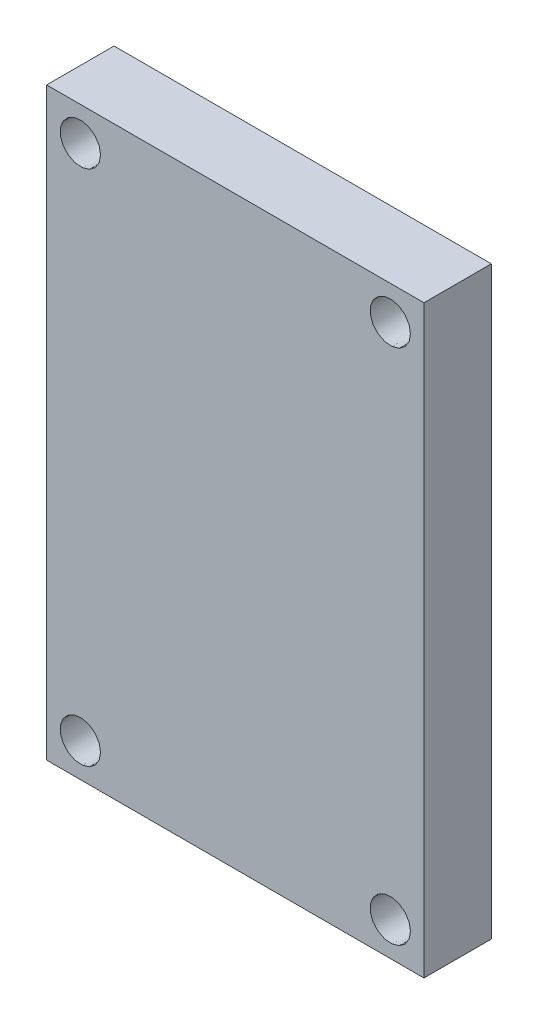
# Autodesk Inventor part: GA010
Saved by Autodesk Inventor 2017 SP1 (Build 210196100, 196)
## iProperties
Created: 2017-06-21
Part Number: GA010
Material: ABS Plastic
Document SubType Name: Modeling
Designer: Zach
Density: 1.06 g/cm^3
Appearance: CR White
Author: Zach
Autodesk Inventor part; units mm, degrees
ref_plane "YZ Plane" through (0, 0, 0) normal (1, 0, 0) x (0, 1, 0)
ref_plane "XZ Plane" through (0, 0, 0) normal (0, 1, 0) x (-1, 0, 0)
ref_plane "XY Plane" through (0, 0, 0) normal (0, 0, 1) x (1, 0, 0)
sketch "Sketch1" plane through (0, 0, 0) normal (0, 0, 1) x (1, 0, 0)
  line L0 (0, 0) -> (28, 0)
  line L1 (28, 0) -> (28, 43.4)
  line L2 (28, 43.4) -> (0, 43.4)
  line L3 (0, 43.4) -> (0, 0)
  line L4 (2.5, 40.9) -> (25.5, 40.9) construction
  line L5 (25.5, 40.9) -> (25.5, 2.5) construction
  line L6 (25.5, 2.5) -> (2.5, 2.5) construction
  line L7 (2.5, 2.5) -> (2.5, 40.9) construction
  circle A0 centre (2.5, 40.9) radius 1.5
  circle A1 centre (25.5, 40.9) radius 1.5
  circle A2 centre (25.5, 2.5) radius 1.5
  circle A3 centre (2.5, 2.5) radius 1.5
  dimension "d0" = 28
  dimension "d1" = 43.4
  dimension "d2" = 2.5
  dimension "d3" = 3
  dimension "d4" = 3
  dimension "d5" = 3
  dimension "d6" = 3
  constraints: 16 end point, 4 centre point, 4 coincident, 4 parallel, 2 perpendicular, 1 horizontal, 3 other
  measures "d0" distance of L2.end L1.end
  measures "d1" distance of L1.end L0.end
  measures "d2" distance between parallel lines of L2 L4
  measures "d3" diameter of A0
  measures "d4" diameter of A1
  measures "d5" diameter of A2
  measures "d6" diameter of A3
extrude "Extrusion1" add sketch "Sketch1" along normal blind 5
body "Solid1"
